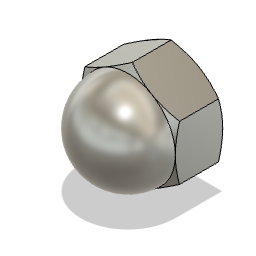
Pendulum (Autodesk Fusion 360 archive; units mm, degrees)
design "Cap Nut NF E27-453 - M6 Steel 6 Plain"
description: Cap Nut NF E27-453 - M6
part number: NF E27-453 - M6 Steel 6 Plain
Autodesk Fusion 360 part; units mm, degrees
sketch "Sketch1" plane through (0, 0, 0) normal (0, 1, 0) x (1, 0, 0)
  line L0 (0, 0) -> (0, -10)
  line L1 (-3, 0) -> (-5, 0)
  line L2 (-5.775, -0.4474) -> (-5.775, -4.5526)
  line L3 (-5.775, -4.5526) -> (-5, -5)
  line L4 (-5.775, -0.4474) -> (-5, 0)
  line L5 (-3, 0) -> (-3, -7.0679)
  line L6 (-3, -7.0679) -> (0, -8.8)
  arc A0 (-5, -5) -> (0, -10) centre (0, -5) ccw
  dimension "d81" = 11.55
  dimension "d145" = 30
  dimension "d147" = 10
  dimension "d148" = 6
  dimension "d150" = 1.2
  dimension "d152" = 10
  dimension "d157" = 30
  dimension "d158" = 5
  dimension "d159" = 30
  constraint coincident L0.start L1
  constraint vertical L0
  constraint parallel L0 L2
  constraint perpendicular L0 L1
  constraint coincident L0.start origin
  constraint vertical L3.end L1.end
  constraint coincident L0 L6.end
  constraint coincident L3 A0.start
  constraint coincident L3.end A0.start
  constraint coincident L0 A0.centre
  measures "d145" angle of L1 L4
  measures "d150" distance of L0.end L6.end
  measures "d152" distance of L1 L0.end
  measures "d157" angle of L1 L6
  measures "d158" distance of L1 L3.end
  measures "d159" angle of L1 L3
revolve "Revolve1" add sketch "Sketch1" angle 360 about axis through (0, 0, 0) along (0, 0, 1)
sketch "Sketch8" plane through (0, 0, 0) normal (0, 0, 1) x (1, 0, 0)
  circle A0 centre (0, 0) radius 5.775
  line L0 (0, 0) -> (-5, 0) construction
  line L1 (-5, 2.8897) -> (-5, -2.8897)
  dimension "d162" = 5
  constraint coincident A0.centre L0.start
  constraint horizontal L0
  constraint coincident A0 L1.start
  constraint coincident A0 L1.end
  constraint perpendicular L0 L1
  constraint coincident L0.end L1
  measures "d162" distance of A0.centre L1
extrude "Extrude5" cut sketch "Sketch8" along normal blind 5 contours A0 L1 picked at (-5.125, 0.7039)
pattern_circular "C-Pattern2" count 6 over 360 about axis through (0, 0, 1.75) along (0, 0, 1) of "Extrude5"
thread "Thread4" "ISO Metric profile 6.0 M6x1 6H" major diameter 6.147 minor diameter 5.035 pitch 1 angle 60 resizes the face on face at (-2.9963, 0.1495, 2.356)
equation "adsk_baseh = 5.00 mm"
equation "adsk_maxdia = 11.55 mm"
equation "adsk_nomdia = 6.00 mm"
equation "d81 = adsk_maxdia"
equation "d89 = adsk_baseh"
equation "adsk_waflat = 10.00 mm"
equation "adsk_nheig = 10.00 mm"
equation "adsk_caprad = 5.00 mm"
equation "adsk_chamang1 = 30.00 deg"
equation "adsk_chamang2 = 30.00 deg"
equation "d145 = adsk_chamang1"
equation "d147 = adsk_waflat"
equation "d148 = adsk_nomdia"
equation "d150 = adsk_nomdia / 5"
equation "d152 = adsk_nheig"
equation "d158 = adsk_baseh"
equation "d162 = adsk_waflat * 0.5"

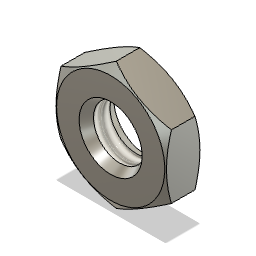
design "Hexagon Thin Nut DIN 439-2 - M4 x 0.7 Steel 6 Plain"
description: Hexagon Thin Nut DIN 439-2 - M4 x 0.7
part number: DIN 439-2 - M4 x 0.7 Steel 6 Plain
Autodesk Fusion 360 part; units mm, degrees
sketch "Sketch1" plane through (0, 0, 0) normal (0, 1, 0) x (1, 0, 0)
  line L0 (0, 0) -> (0, -2.2)
  line L1 (-2, 0) -> (-3.43, 0)
  line L2 (-3.43, 0) -> (-4.0425, -0.3536)
  line L3 (-4.0425, -0.3536) -> (-4.0425, -1.8464)
  line L4 (-4.0425, -1.8464) -> (-3.43, -2.2)
  line L5 (-3.43, -2.2) -> (-2, -2.2)
  line L6 (-2, -2.2) -> (-2, 0)
  dimension "d121" = 4
  dimension "d122" = 30
  dimension "d123" = 30
  dimension "d126" = 2.2
  dimension "d128" = 8.085
  dimension "d172" = 6.86
  constraint vertical L0
  constraint coincident L0 L0.end
  constraint coincident origin L0
  constraint horizontal L1
  constraint perpendicular L1 L3
  constraint perpendicular L3 L5
  constraint perpendicular L5 L6
  constraint coincident L0.start L1
  constraint coincident L0.start origin
  constraint coincident L0.end L5
  constraint vertical L1.end L4.end
  measures "d122" angle of L1 L2
  measures "d123" angle of L4 L5
  measures "d126" distance of L1.start L5.end
revolve "Revolve1" add sketch "Sketch1" angle 360 about axis through (0, 0, 0) along (0, 0, 1)
sketch "Sketch8" plane through (0, 0, 2.2) normal (0, 0, 1) x (1, 0, 0)
  line L0 (0, 0) -> (-7, 0) construction
  line L1 (-3.5, -2.0228) -> (-3.5, 2.0228)
  circle A0 centre (0, 0) radius 2
  circle A1 centre (0, 0) radius 4.0425
  dimension "d114" = 3.5
  constraint horizontal L0
  constraint perpendicular L0 L1
  constraint midpoint L0 L1
  constraint coincident L0.start A0.centre
  constraint coincident L1.end A1
  measures "d114" distance of L0.start L1
extrude "Extrude5" cut sketch "Sketch8" against normal blind 2.2 contours L1 A1 picked at (-3.5875, -0.4927)
pattern_circular "C-Pattern2" count 6 over 360 about axis through (0, 0, 1.75) along (0, 0, 1) of "Extrude5"
thread "Thread3" "ISO Metric profile 4.0 M4x0.7 6H" major diameter 4.1095 minor diameter 3.332 pitch 0.7 angle 60 resizes the face on face at (-1.9901, 0.1991, 1.4667)
sketch "Sketch12" plane through (0, 0, 0) normal (0, 1, 0) x (1, 0, 0)
  line L0 (1.666, -2.2) -> (-1.666, -2.2)
  line L1 (3.43, -2.2) -> (-3.43, -2.2)
  line L2 (3.43, 0) -> (-3.43, 0)
  line L3 (1.666, 0) -> (-1.666, 0)
  line L4 (-2, 0) -> (0, 0)
  line L5 (-1.3649, -1.1) -> (-2, 0)
  line L6 (-2, -2.2) -> (0, -2.2)
  line L7 (-1.3649, -1.1) -> (-2, -2.2)
  line L8 (0, 0) -> (0, -2.2)
  dimension "d165" = 60
  dimension "d169" = 60
  dimension "d170" = 2
  constraint horizontal L4
  constraint collinear L1 L6
  constraint coincident L5.start L7.start
  constraint vertical L4.start L6.start
  constraint coincident L1 L6.end
  constraint coincident L6.end L8.end
  constraint coincident L4.end L8.start
  measures "d165" angle of L2 L5
  measures "d169" angle of L6 L7
  measures "d170" distance of L4.start L4.end
revolve "Revolve3" cut sketch "Sketch12" angle 360 about axis through (0, 0, 1.75) along (0, 0, 1)
equation "adsk_nheig = 2.20 mm"
equation "adsk_maxdia = 8.085 mm"
equation "adsk_nomdia = 4.00 mm"
equation "d89 = -adsk_nheig"
equation "adsk_waflat = 7.00 mm"
equation "d114 = adsk_waflat / 2"
equation "adsk_chamang1 = 30.00 deg"
equation "adsk_chamang2 = 30.00 deg"
equation "d121 = adsk_nomdia"
equation "d122 = adsk_chamang1"
equation "d123 = adsk_chamang2"
equation "d126 = adsk_nheig"
equation "d128 = adsk_maxdia"
equation "d163 = adsk_nheig"
equation "d170 = adsk_nomdia * 0.5"
equation "adsk_beardia = 6.86 mm"
equation "d172 = adsk_beardia"

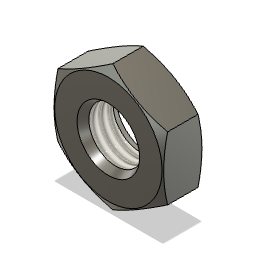
design "Hex Jam Nut ANSI B18.2.2 - 1/4-28 Steel Grade 2H Plain"
description: Hex Jam Nut ANSI B18.2.2 - 1/4-28
part number: HJN ANSI B18.2.2 - 1/4-28 Steel Grade 2H Plain
Autodesk Fusion 360 part; units mm, degrees
sketch "Sketch1" plane through (0, 0, 0) normal (0, 1, 0) x (1, 0, 0)
  line L0 (0, 0) -> (0, -3.9878)
  line L1 (-3.175, 0) -> (-5.4513, 0)
  line L2 (-5.4513, 0) -> (-6.4248, -0.4539)
  line L3 (-6.4248, -0.4539) -> (-6.4248, -3.5339)
  line L4 (-6.4248, -3.5339) -> (-5.4513, -3.9878)
  line L5 (-5.4513, -3.9878) -> (-3.175, -3.9878)
  line L6 (-3.175, -3.9878) -> (-3.175, 0)
  line L7 (-5.4513, -3.9878) -> (-5.4513, 0) construction
  dimension "d121" = 6.35
  dimension "d122" = 25
  dimension "d123" = 25
  dimension "d126" = 3.9878
  dimension "d128" = 12.8496
  dimension "d170" = 10.9027
  constraint vertical L0
  constraint coincident L0 L0.end
  constraint coincident origin L0
  constraint horizontal L1
  constraint perpendicular L1 L3
  constraint perpendicular L3 L5
  constraint perpendicular L5 L6
  constraint coincident L0.start L1
  constraint coincident L0.end L5
  constraint coincident L0.start origin
  constraint vertical L7
  measures "d122" angle of L1 L2
  measures "d123" angle of L4 L5
  measures "d126" distance of L1.start L5.end
revolve "Revolve1" add sketch "Sketch1" angle 360 about axis through (0, 0, 0) along (0, 0, 1)
sketch "Sketch8" plane through (0, 0, 3.9878) normal (0, 0, 1) x (1, 0, 0)
  line L0 (0, 0) -> (-11.1252, 0) construction
  line L1 (-5.5626, -3.2149) -> (-5.5626, 3.2149)
  circle A0 centre (0, 0) radius 3.175
  circle A1 centre (0, 0) radius 6.4248
  dimension "d114" = 5.5626
  constraint horizontal L0
  constraint perpendicular L0 L1
  constraint midpoint L0 L1
  constraint coincident L0.start A0.centre
  constraint coincident L1.end A1
  measures "d114" distance of L0.start L1
extrude "Extrude5" cut sketch "Sketch8" against normal blind 3.9878 contours L1 A1 picked at (-5.7017, 0.7831)
pattern_circular "C-Pattern2" count 6 over 360 about axis through (0, 0, 1.75) along (0, 0, 1) of "Extrude5"
thread "Thread3" "ANSI Unified Screw Threads 0.25 1/4-28 UNF 2B" major diameter 6.35 minor diameter 5.4737 pitch 0.9071 angle 60 resizes the face on face at (-3.1711, 0.1583, 2.6585)
sketch "Sketch12" plane through (0, 0, 0) normal (0, 1, 0) x (1, 0, 0)
  line L0 (0, 0) -> (-3.175, 0)
  line L1 (0, 0) -> (0, -3.9878)
  line L2 (0, -3.9878) -> (-3.175, -3.9878)
  line L3 (-3.175, -3.9878) -> (-2.0238, -1.9939)
  line L4 (-3.175, 0) -> (-2.0238, -1.9939)
  dimension "d164" = 60
  dimension "d165" = 60
  dimension "d166" = 3.175
  constraint coincident L0.start L1.start
  constraint horizontal L0
  constraint coincident L1.end L2.start
  constraint perpendicular L1 L2
  constraint vertical L0.end L2.end
  constraint coincident L3.end L4.end
  measures "d164" angle of L0 L4
  measures "d165" angle of L2 L3
  measures "d166" distance of L0.start L0.end
revolve "Revolve3" cut sketch "Sketch12" angle 360 about axis through (0, 0, 1.75) along (0, 0, 1)
equation "d89 = -adsk_nheig"
equation "d114 = adsk_waflat / 2"
equation "adsk_chamang1 = 25.00 deg"
equation "adsk_chamang2 = 25.00 deg"
equation "d121 = adsk_nomdia"
equation "d122 = adsk_chamang1"
equation "d123 = adsk_chamang2"
equation "d126 = adsk_nheig"
equation "d128 = adsk_maxdia"
equation "adsk_nheig = 0.157 in"
equation "adsk_maxdia = 0.50589 in"
equation "adsk_nomdia = 0.25 in"
equation "adsk_waflat = 0.438 in"
equation "d162 = adsk_nheig"
equation "d166 = adsk_nomdia * 0.50"
equation "adsk_beardia = adsk_waflat * 0.98"
equation "d170 = adsk_beardia"

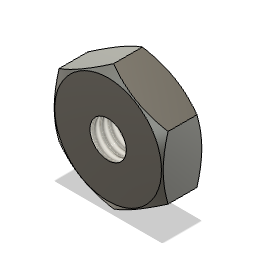
design "Chamfered Bottom Hex Machine Screw Nut ASME B18.6.3 - 5-44 Steel Grade 2H Plain"
description: Chamfered Bottom Hex Machine Screw Nut ASME B18.6.3 - 5-44
part number: CBHMSN ASME B18.6.3 - 5-44 Steel Grade 2H Plain
Autodesk Fusion 360 part; units mm, degrees
sketch "Sketch1" plane through (0, 0, 0) normal (0, 1, 0) x (1, 0, 0)
  line L0 (0, 0) -> (0, -2.8956)
  line L1 (-1.5875, 0) -> (-3.8832, 0)
  line L2 (-3.8832, 0) -> (-4.5847, -0.405)
  line L3 (-4.5847, -0.405) -> (-4.5847, -2.4906)
  line L4 (-4.5847, -2.4906) -> (-3.8832, -2.8956)
  line L5 (-3.8832, -2.8956) -> (-1.5875, -2.8956)
  line L6 (-1.5875, -2.8956) -> (-1.5875, 0)
  dimension "d121" = 3.175
  dimension "d122" = 30
  dimension "d123" = 30
  dimension "d126" = 2.8956
  dimension "d128" = 9.1694
  dimension "d142" = 7.7663
  constraint vertical L0
  constraint coincident L0 L0.end
  constraint coincident origin L0
  constraint horizontal L1
  constraint perpendicular L1 L3
  constraint perpendicular L3 L5
  constraint perpendicular L5 L6
  constraint coincident L0.start L1
  constraint coincident L0.start origin
  constraint vertical L1.end L4.end
  constraint coincident L0.end L5
  measures "d122" angle of L1 L2
  measures "d123" angle of L4 L5
  measures "d126" distance of L1.start L5.end
revolve "Revolve1" add sketch "Sketch1" angle 360 about axis through (0, 0, 0) along (0, 0, 1)
sketch "Sketch8" plane through (0, 0, 2.8956) normal (0, 0, 1) x (1, 0, 0)
  line L0 (0, 0) -> (-7.9248, 0) construction
  line L1 (-3.9624, -2.3063) -> (-3.9624, 2.3063)
  circle A0 centre (0, 0) radius 1.5875
  circle A1 centre (0, 0) radius 4.5847
  dimension "d114" = 3.9624
  constraint horizontal L0
  constraint perpendicular L0 L1
  constraint midpoint L0 L1
  constraint coincident L0.start A0.centre
  constraint coincident L1.end A1
  measures "d114" distance of L0.start L1
extrude "Extrude5" cut sketch "Sketch8" against normal blind 2.8956 contours L1 A1 picked at (-4.052, 0.5885)
pattern_circular "C-Pattern2" count 6 over 360 about axis through (0, 0, 1.75) along (0, 0, 1) of "Extrude5"
thread "Thread3" "ANSI Unified Screw Threads 0.125(#5) 5-44 UNF 2B" major diameter 3.175 minor diameter 2.6467 pitch 0.5773 angle 60 resizes the face on face at (-1.5855, 0.0791, 1.9304)
equation "d89 = -adsk_nheig"
equation "d114 = adsk_waflat / 2"
equation "adsk_chamang1 = 30 deg"
equation "adsk_chamang2 = 30 deg"
equation "d121 = adsk_nomdia"
equation "d122 = adsk_chamang1"
equation "d123 = adsk_chamang2"
equation "d126 = adsk_nheig"
equation "d128 = adsk_maxdia"
equation "adsk_nheig = 0.114 in"
equation "adsk_maxdia = 0.361 in"
equation "adsk_nomdia = 0.125 in"
equation "adsk_waflat = 0.312 in"
equation "d139 = adsk_nheig"
equation "adsk_beardia = adsk_waflat * 0.98"
equation "d142 = adsk_beardia"

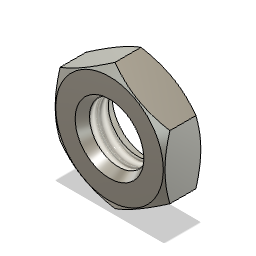
design "Hexagon Thin Nut DIN 439-2 - M5 x 0.8 Steel 6 Plain"
description: Hexagon Thin Nut DIN 439-2 - M5 x 0.8
part number: DIN 439-2 - M5 x 0.8 Steel 6 Plain
Autodesk Fusion 360 part; units mm, degrees
sketch "Sketch1" plane through (0, 0, 0) normal (0, 1, 0) x (1, 0, 0)
  line L0 (0, 0) -> (0, -2.7)
  line L1 (-2.5, 0) -> (-3.92, 0)
  line L2 (-3.92, 0) -> (-4.62, -0.4041)
  line L3 (-4.62, -0.4041) -> (-4.62, -2.2959)
  line L4 (-4.62, -2.2959) -> (-3.92, -2.7)
  line L5 (-3.92, -2.7) -> (-2.5, -2.7)
  line L6 (-2.5, -2.7) -> (-2.5, 0)
  dimension "d121" = 5
  dimension "d122" = 30
  dimension "d123" = 30
  dimension "d126" = 2.7
  dimension "d128" = 9.24
  dimension "d172" = 7.84
  constraint vertical L0
  constraint coincident L0 L0.end
  constraint coincident origin L0
  constraint horizontal L1
  constraint perpendicular L1 L3
  constraint perpendicular L3 L5
  constraint perpendicular L5 L6
  constraint coincident L0.start L1
  constraint coincident L0.start origin
  constraint coincident L0.end L5
  constraint vertical L1.end L4.end
  measures "d122" angle of L1 L2
  measures "d123" angle of L4 L5
  measures "d126" distance of L1.start L5.end
revolve "Revolve1" add sketch "Sketch1" angle 360 about axis through (0, 0, 0) along (0, 0, 1)
sketch "Sketch8" plane through (0, 0, 2.7) normal (0, 0, 1) x (1, 0, 0)
  line L0 (0, 0) -> (-8, 0) construction
  line L1 (-4, -2.3118) -> (-4, 2.3118)
  circle A0 centre (0, 0) radius 2.5
  circle A1 centre (0, 0) radius 4.62
  dimension "d114" = 4
  constraint horizontal L0
  constraint perpendicular L0 L1
  constraint midpoint L0 L1
  constraint coincident L0.start A0.centre
  constraint coincident L1.end A1
  measures "d114" distance of L0.start L1
extrude "Extrude5" cut sketch "Sketch8" against normal blind 2.7 contours L1 A1 picked at (-4.1, -0.5631)
pattern_circular "C-Pattern2" count 6 over 360 about axis through (0, 0, 1.75) along (0, 0, 1) of "Extrude5"
thread "Thread3" "ISO Metric profile 5.0 M5x0.8 6H" major diameter 5.12 minor diameter 4.234 pitch 0.8 angle 60 resizes the face on face at (-2.4969, 0.1246, 1.8)
sketch "Sketch12" plane through (0, 0, 0) normal (0, 1, 0) x (1, 0, 0)
  line L0 (2.117, -2.7) -> (-2.117, -2.7)
  line L1 (3.92, -2.7) -> (-3.92, -2.7)
  line L2 (3.92, 0) -> (-3.92, 0)
  line L3 (2.117, 0) -> (-2.117, 0)
  line L4 (-2.5, 0) -> (0, 0)
  line L5 (-1.7206, -1.35) -> (-2.5, 0)
  line L6 (-2.5, -2.7) -> (0, -2.7)
  line L7 (-1.7206, -1.35) -> (-2.5, -2.7)
  line L8 (0, 0) -> (0, -2.7)
  dimension "d165" = 60
  dimension "d169" = 60
  dimension "d170" = 2.5
  constraint horizontal L4
  constraint collinear L1 L6
  constraint coincident L5.start L7.start
  constraint vertical L4.start L6.start
  constraint coincident L1 L6.end
  constraint coincident L6.end L8.end
  constraint coincident L4.end L8.start
  measures "d165" angle of L2 L5
  measures "d169" angle of L6 L7
  measures "d170" distance of L4.start L4.end
revolve "Revolve3" cut sketch "Sketch12" angle 360 about axis through (0, 0, 1.75) along (0, 0, 1)
equation "adsk_nheig = 2.70 mm"
equation "adsk_maxdia = 9.24 mm"
equation "adsk_nomdia = 5.00 mm"
equation "d89 = -adsk_nheig"
equation "adsk_waflat = 8.00 mm"
equation "d114 = adsk_waflat / 2"
equation "adsk_chamang1 = 30.00 deg"
equation "adsk_chamang2 = 30.00 deg"
equation "d121 = adsk_nomdia"
equation "d122 = adsk_chamang1"
equation "d123 = adsk_chamang2"
equation "d126 = adsk_nheig"
equation "d128 = adsk_maxdia"
equation "d163 = adsk_nheig"
equation "d170 = adsk_nomdia * 0.5"
equation "adsk_beardia = 7.84 mm"
equation "d172 = adsk_beardia"
